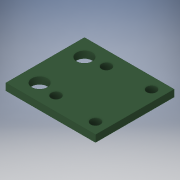
# Autodesk Inventor part: ACHS-7121
Saved by Autodesk Inventor 2019 (Build 230136000, 136)
## iProperties
Created: 2019-10-11
Part Number: ACHS-7121
Material: Generic
Document SubType Name: Modeling
Designer: james
Density: 1 g/cm^3
Appearance: Default(1)
Author: james
Autodesk Inventor part; units mm, degrees
ref_plane "YZ Plane" through (0, 0, 0) normal (1, 0, 0) x (0, 1, 0)
ref_plane "XZ Plane" through (0, 0, 0) normal (0, 1, 0) x (-1, 0, 0)
ref_plane "XY Plane" through (0, 0, 0) normal (0, 0, 1) x (1, 0, 0)
sketch "Sketch1" plane through (0, 0, 0) normal (0, 1, 0) x (-1, 0, 0)
  line L0 (12.6186, 12.1817) -> (-7.6814, 12.1817)
  line L1 (-7.6814, 12.1817) -> (-7.6814, -5.6183)
  line L2 (-7.6814, -5.6183) -> (12.6186, -5.6183)
  line L3 (12.6186, -5.6183) -> (12.6186, 12.1817)
  point P0 (0, 0)
  dimension "d0" = 17.8
  dimension "d1" = 20.3
  constraints: 8 end point, 2 parallel, 1 horizontal, 1 perpendicular
  measures "d0" distance of L2.end L0.start
  measures "d1" distance of L0.start L0.end
extrude "Extrusion1" add sketch "Sketch1" along normal blind 1.57
sketch "Sketch2" plane through (0, 1.57, 0) normal (0, 1, 0) x (1, 0, 0)
  circle A0 centre (-8.8086, -8.3717) radius 1.78
  circle A1 centre (-8.8086, 1.7883) radius 1.78
  circle A2 centre (-4.4586, -9.0017) radius 1.09
  circle A3 centre (-4.4586, 2.4283) radius 1.09
  circle A4 centre (5.1814, 3.0183) radius 1.09
  circle A5 centre (5.1814, -9.6817) radius 1.09
  line L0 (-12.6186, 5.6183) -> (-12.6186, -12.1817) projected
  line L1 (-12.6186, -12.1817) -> (7.6814, -12.1817) projected
  line L2 (7.6814, -12.1817) -> (7.6814, 5.6183) projected
  point P0 (0, 0)
  dimension "d4" = 3.56
  dimension "d5" = 3.56
  dimension "d6" = 3.81
  dimension "d7" = 3.81
  dimension "d8" = 3.81
  dimension "d9" = 10.16
  dimension "d10" = 2.18
  dimension "d11" = 2.18
  dimension "d12" = 2.18
  dimension "d13" = 2.18
  dimension "d14" = 8.16
  dimension "d15" = 8.16
  dimension "d16" = 3.18
  dimension "d17" = 11.43
  dimension "d18" = 2.5
  dimension "d19" = 2.5
  dimension "d20" = 12.7
  dimension "d21" = 2.5
  constraints: 6 centre point
  measures "d4" diameter of A0
  measures "d5" diameter of A1
  measures "d6" distance from line of L0 A0.centre
  measures "d7" distance from line of L0 A1.centre
  measures "d8" distance from line of L1 A0.centre
  measures "d9" distance of A1.centre A0.centre
  measures "d10" diameter of A2
  measures "d11" diameter of A3
  measures "d12" diameter of A4
  measures "d13" diameter of A5
  measures "d14" distance from line of L0 A2.centre
  measures "d15" distance from line of L0 A3.centre
  measures "d16" distance from line of L1 A2.centre
  measures "d17" distance of A2.centre A3.centre
  measures "d18" distance from line of L2 A5.centre
  measures "d19" distance from line of L1 A5.centre
  measures "d20" distance of A4.centre A5.centre
  measures "d21" distance from line of L2 A4.centre
extrude "Extrusion2" cut sketch "Sketch2" against normal blind 50.8
body "Solid1"
